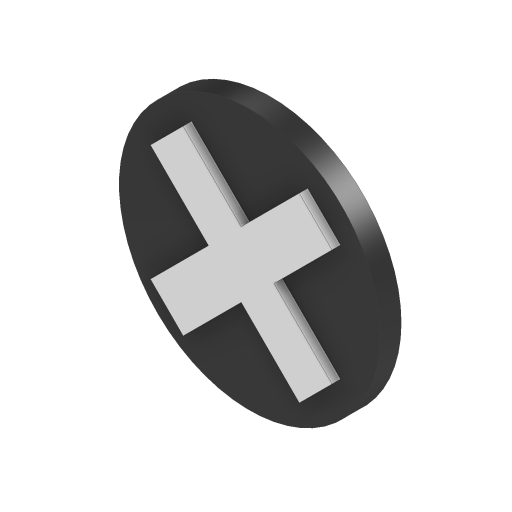
# Autodesk Inventor part: button_plate_cross
Saved by Autodesk Inventor 2023 (Build 270158000, 158)
## iProperties
Created: 2025-02-19
Part Number: button_plate_cross
Material: Všeobecné
Document SubType Name: Modeling
Designer: Marek
Density: 1 g/cm^3
Appearance: Výchozí
Author: Marek
Autodesk Inventor part; units mm, degrees
ref_plane "YZ Plane" through (0, 0, 0) normal (1, 0, 0) x (0, 1, 0)
ref_plane "XZ Plane" through (0, 0, 0) normal (0, 1, 0) x (-1, 0, 0)
ref_plane "XY Plane" through (0, 0, 0) normal (0, 0, 1) x (1, 0, 0)
sketch "Náčrt1" plane through (0, 0, 0) normal (0, 0, 1) x (1, 0, 0)
  line L0 (0, 8.68) -> (0, -8.68) projected
  line L1 (-8.68, 0) -> (8.68, 0) projected
  circle A0 centre (0, 0) radius 6.2
  dimension "d0" = 12.4
  constraints: 1 centre point, 1 coincident
  measures "d0" diameter of A0
extrude "Vysunutí1" add sketch "Náčrt1" along normal blind 1
sketch "Náčrt2" plane through (0, 0, 1) normal (0, 0, 1) x (1, 0, 0)
  line L0 (-8.68, 0) -> (8.68, 0) projected
  line L1 (0, 8.68) -> (0, -8.68) projected
  line L2 (0, 1.5556) -> (-2.7577, 4.3134)
  line L3 (-2.7577, 4.3134) -> (-4.3134, 2.7577)
  line L4 (-4.3134, 2.7577) -> (-1.5556, 0)
  line L5 (0, 0) -> (-4.3841, 4.3841)
  circle A0 centre (0, 0) radius 6.2 projected
  line L6 (0, 0) -> (6.2, 0) construction
  line L7 (-4.3134, -2.7577) -> (-2.7577, -4.3134)
  line L8 (-1.5556, 0) -> (-4.3134, -2.7577)
  line L9 (-2.7577, -4.3134) -> (0, -1.5556)
  line L10 (2.7577, -4.3134) -> (4.3134, -2.7577)
  line L11 (0, -1.5556) -> (2.7577, -4.3134)
  line L12 (4.3134, -2.7577) -> (1.5556, 0)
  line L13 (4.3134, 2.7577) -> (2.7577, 4.3134)
  line L14 (1.5556, 0) -> (4.3134, 2.7577)
  line L15 (2.7577, 4.3134) -> (0, 1.5556)
  point P0 (-1.5556, 0)
  point P1 (0, -1.5556)
  point P2 (1.5556, 0)
  dimension "d3" = 2.2
  dimension "d4" = 5
  dimension "d5" = 135
  dimension "d8" = 360
  constraints: 28 end point, 2 perpendicular, 2 point on line, 1 equal length, 1 horizontal, 32 other
  measures "d3" distance between parallel lines of L4 L2
  measures "d4" distance from line of L5.start L3
  measures "d5" angle of L6 L5
extrude "Vysunutí2" add sketch "Náčrt2" along normal blind 0.4 contours L4 L3 L5 L0 | L0 L1 L9 L7 L8 | L1 L15 L13 L14 L0 | L5 L3 L2 L1 | L0 L12 L10 L11 L1
